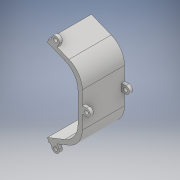
# Autodesk Inventor part: Capture Zone4
Saved by Autodesk Inventor 2018 (Build 220112000, 112)
## iProperties
Created: 2017-10-23
Part Number: Capture Zone4
Material: Generic
Document SubType Name: Modeling
Designer: BrisbaneMatt
Density: 1 g/cm^3
Appearance: Default
Author: BrisbaneMatt
Autodesk Inventor part; units mm, degrees
ref_plane "YZ Plane" through (0, 0, 0) normal (1, 0, 0) x (0, 1, 0)
ref_plane "XZ Plane" through (0, 0, 0) normal (0, 1, 0) x (-1, 0, 0)
ref_plane "XY Plane" through (0, 0, 0) normal (0, 0, 1) x (1, 0, 0)
sketch "Sketch1" plane through (0, 0, 0) normal (0, 1, 0) x (-1, 0, 0)
  line L0 (0, 0) -> (0, -54.7595)
  line L1 (0, -54.7595) -> (17.2816, -61.6681)
  line L2 (0, -54.7595) -> (18.6114, -54.7595) construction
  line L3 (0, -54.7595) -> (28.8848, -66.3067)
  line L4 (28.8848, -66.3067) -> (28.8848, -54.7595)
  line L5 (28.8848, -54.7595) -> (28.8848, 0)
  line L6 (28.8848, 0) -> (28.8848, 11.5473)
  line L7 (28.8848, 11.5473) -> (0, 0)
  line L8 (0, -50.5358) -> (-4, -50.5358)
  line L9 (3.9418, -56.3353) -> (2.457, -60.0495)
  line L10 (2.457, -60.0495) -> (-4, -57.4682)
  line L11 (-4, -57.4682) -> (-4, -50.5358)
  line L12 (28.8848, -66.3067) -> (27.4, -70.0209)
  line L13 (27.4, -70.0209) -> (2.457, -60.0495)
  line L14 (0, -3.5872) -> (-4, -3.5872)
  line L15 (-4, -3.5872) -> (-4, -50.5358)
  line L16 (2.457, 0.9822) -> (0.9721, 4.6964)
  line L17 (0.9721, 4.6964) -> (-4, 2.7087)
  line L18 (-4, 2.7087) -> (-4, -3.5872)
  line L19 (23.3647, 9.3405) -> (21.8799, 13.0547)
  line L20 (21.8799, 13.0547) -> (0.9721, 4.6964)
  line L21 (28.8848, 11.5473) -> (27.4, 15.2615)
  line L22 (27.4, 15.2615) -> (21.8799, 13.0547)
  dimension "d0" = 54.7595
  dimension "d1" = 21.79
  dimension "d2" = 31.1075
  dimension "d3" = 11.5473
  dimension "d4" = 11.5473
  dimension "d5" = 4
  dimension "d6" = 4
  dimension "d7" = 4
  constraints: 46 end point, 12 perpendicular, 11 point on line, 4 vertical, 1 collinear, 1 equal length, 1 horizontal
  measures "d0" distance of L0.start L0.end
  measures "d1" angle of L1 L2
  measures "d2" distance of L0.end L3.end
  measures "d3" distance of L3.end L4.end
  measures "d4" distance of L5.end L6.end
  measures "d5" distance of L8.start L8.end
  measures "d6" distance of L9.start L9.end
  measures "d7" distance of L16.start L16.end
extrude "Extrusion1" add sketch "Sketch1" along normal blind 40 contours L0 L14 L18 L17 L16 L7 | L0 L8 L15 L14 | L16 L20 L19 L7 | L0 L1 L9 L10 L11 L8 | L19 L22 L21 L7 | L1 L3 L12 L13 L9
sketch "Sketch2" plane through (0, 0, 0) normal (0, -1, 0) x (1, 0, 0)
  line L0 (0, -54.7595) -> (0, 0) projected
  line L1 (0, -27.3797) -> (8, -27.3797)
  circle A0 centre (8, -27.3797) radius 1.75
  circle A1 centre (8, -27.3797) radius 3.5
  line L2 (4, 2.7087) -> (4, -57.4682) projected
  line L3 (4, -27.3797) -> (4, -30.8797)
  line L4 (4, -30.8797) -> (8, -30.8797)
  line L5 (4, -27.3797) -> (4, -23.8797)
  line L6 (4, -23.8797) -> (8, -23.8797)
  line L7 (-27.4, -70.0209) -> (-28.8848, -66.3067) projected
  line L8 (-28.8848, -66.3067) -> (-27.0288, -70.9495)
  line L9 (-27.0288, -70.9495) -> (-28.8848, -66.3067)
  line L10 (-28.8848, -66.3067) -> (-24.2421, -64.4507)
  line L11 (-24.2421, -64.4507) -> (-21.2724, -71.8791)
  circle A2 centre (-21.2724, -71.8791) radius 1.75
  circle A3 centre (-21.2724, -71.8791) radius 3.5
  line L12 (4, -57.4682) -> (-27.4, -70.0209) projected
  line L13 (-22.7573, -68.1649) -> (-26.0072, -69.4641)
  line L14 (-26.0072, -69.4641) -> (-24.5224, -73.1783)
  line L15 (-22.7573, -68.1649) -> (-19.5073, -66.8657)
  line L16 (-19.5073, -66.8657) -> (-18.0225, -70.5799)
  line L17 (-28.8848, 11.5473) -> (-24.2421, 9.6912)
  line L18 (0, 0) -> (-28.8848, 11.5473) projected
  line L19 (-24.2421, 9.6912) -> (-21.2724, 17.1196)
  circle A4 centre (-21.2724, 17.1196) radius 1.75
  circle A5 centre (-21.2724, 17.1196) radius 3.5
  line L20 (-27.4, 15.2615) -> (4, 2.7087) projected
  line L21 (-22.7573, 13.4054) -> (-26.0072, 14.7047)
  line L22 (-26.0072, 14.7047) -> (-24.5224, 18.4189)
  line L23 (-22.7573, 13.4054) -> (-19.5073, 12.1062)
  line L24 (-19.5073, 12.1062) -> (-18.0225, 15.8204)
  dimension "d10" = 8
  dimension "d11" = 3.5
  dimension "d12" = 7
  dimension "d13" = 5
  dimension "d14" = 5
  dimension "d15" = 8
  dimension "d16" = 3.5
  dimension "d17" = 7
  dimension "d18" = 3.5
  dimension "d19" = 3.5
  dimension "d20" = 5
  dimension "d21" = 3.5
  dimension "d22" = 7
  dimension "d23" = 3.5
  constraints: 38 end point, 9 point on line, 8 perpendicular, 6 centre point, 6 coincident, 6 point on circle, 4 midpoint, 2 collinear, 1 horizontal
  measures "d10" distance of L1.start L1.end
  measures "d11" diameter of A0
  measures "d12" diameter of A1
  measures "d13" distance of L7.end L8.end
  measures "d14" distance of L7.end L10.end
  measures "d15" distance of L10.end L11.end
  measures "d16" diameter of A2
  measures "d17" diameter of A3
  measures "d18" distance of L13.start L13.end
  measures "d19" distance of L13.start L15.end
  measures "d20" distance of L17.start L17.end
  measures "d21" diameter of A4
  measures "d22" diameter of A5
  measures "d23" distance of L21.start L23.end
extrude "Extrusion2" add sketch "Sketch2" against normal blind 3 contours L16 A3 L11 L12 | L2 L6 A1 L1 | L1 A1 L4 L2 | A1 | L20 L22 A5 L19 | L19 A5 L24 L20 | A5 | L11 A3 L14 L12 | A3
sketch "Sketch3" plane through (0, 40, 0) normal (0, 1, 0) x (1, 0, 0)
  line L0 (4, 23.8797) -> (4, 30.8797) projected
  line L1 (4, 27.3797) -> (4, 30.8797)
  line L2 (8, 30.8797) -> (4, 30.8797) projected
  line L3 (4, 30.8797) -> (8, 30.8797)
  line L4 (4, 27.3797) -> (4, 23.8797)
  line L5 (4, 23.8797) -> (8, 23.8797) projected
  line L6 (4, 23.8797) -> (8, 23.8797)
  circle A0 centre (8, 27.3797) radius 1.75 projected
  circle A1 centre (8, 27.3797) radius 1.75
  circle A2 centre (8, 27.3797) radius 3.5
  point P0 (0, 0)
  constraints: 8 end point, 3 collinear, 2 centre point, 2 coincident, 1 midpoint, 1 perpendicular
extrude "Extrusion3" add sketch "Sketch3" against normal blind 3 contours A2
sketch "Sketch4" plane through (0, 40, 0) normal (0, 1, 0) x (1, 0, 0)
  line L0 (4, 23.8797) -> (4, 30.8797) projected
  line L1 (4, 23.8797) -> (8, 23.8797)
  circle A0 centre (8, 27.3797) radius 3.5 projected
  line L2 (8, 30.8797) -> (4, 30.8797) projected
  line L3 (4, 30.8797) -> (8, 30.8797)
  point P0 (0, 0)
  constraints: 4 end point, 1 collinear, 1 horizontal, 1 point on circle
extrude "Extrusion4" add sketch "Sketch4" against normal blind 3 contours L0 L2 A0 L1
sketch "Sketch5" plane through (0, 40, 0) normal (0, 1, 0) x (1, 0, 0)
  point P0 (0, 0)
fillet "Fillet1" radius 20 4 edges at (0, 20, 0) (0, 20, -54.7595) (4, 20, 2.7087) (4, 20, -57.4682)
body "Solid1"
